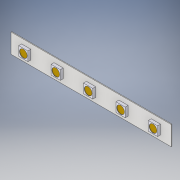
# Autodesk Inventor part: LEDStrip 5x
Saved by Autodesk Inventor 2019 (Build 230136000, 136)
## iProperties
Created: 2022-03-28
Part Number: LEDStrip 5x
Material: Generic
Document SubType Name: Modeling
Designer: Lix
Density: 1 g/cm^3
Appearance: Default
Author: Lix
Autodesk Inventor part; units mm, degrees
ref_plane "YZ Plane" through (0, 0, 0) normal (1, 0, 0) x (0, 1, 0)
ref_plane "XZ Plane" through (0, 0, 0) normal (0, 1, 0) x (-1, 0, 0)
ref_plane "XY Plane" through (0, 0, 0) normal (0, 0, 1) x (1, 0, 0)
sketch "Sketch1" plane through (0, 0, 0) normal (0, 0, 1) x (1, 0, 0)
  line L0 (-41.5, 5) -> (41.5, 5)
  line L1 (41.5, 5) -> (41.5, -5)
  line L2 (41.5, -5) -> (-41.5, -5)
  line L3 (-41.5, -5) -> (-41.5, 5)
  line L4 (-41.5, 5) -> (41.5, -5) construction
  line L5 (41.5, 5) -> (-41.5, -5) construction
  point P0 (0, 0)
  dimension "d0" = 83
  dimension "d1" = 10
  constraints: 12 end point, 2 midpoint, 2 parallel, 1 horizontal, 1 perpendicular
  measures "d0" distance of L1.end L2.end
  measures "d1" distance of L0.end L1.end
extrude "Extrusion1" add sketch "Sketch1" along normal blind 0.4
sketch "Sketch2" plane through (0, 0, 0.4) normal (0, 0, 1) x (1, 0, 0)
  line L0 (31.2, 2.4) -> (36, 2.4)
  line L1 (36, 2.4) -> (36, -2.4)
  line L2 (36, -2.4) -> (31.2, -2.4)
  line L3 (31.2, -2.4) -> (31.2, 2.4)
  line L4 (31.2, 2.4) -> (36, -2.4) construction
  line L5 (36, 2.4) -> (31.2, -2.4) construction
  line L6 (-41.5, 5) -> (-41.5, -5) projected
  line L7 (41.5, -5) -> (41.5, 5) projected
  line L8 (14.4, 2.4) -> (19.2, 2.4)
  line L9 (19.2, 2.4) -> (19.2, -2.4)
  line L10 (19.2, -2.4) -> (14.4, -2.4)
  line L11 (14.4, -2.4) -> (14.4, 2.4)
  line L12 (14.4, 2.4) -> (19.2, -2.4) construction
  line L13 (19.2, 2.4) -> (14.4, -2.4) construction
  line L14 (-2.4, 2.4) -> (2.4, 2.4)
  line L15 (2.4, 2.4) -> (2.4, -2.4)
  line L16 (2.4, -2.4) -> (-2.4, -2.4)
  line L17 (-2.4, -2.4) -> (-2.4, 2.4)
  line L18 (-2.4, 2.4) -> (2.4, -2.4) construction
  line L19 (2.4, 2.4) -> (-2.4, -2.4) construction
  line L20 (-19.2, 2.4) -> (-14.4, 2.4)
  line L21 (-14.4, 2.4) -> (-14.4, -2.4)
  line L22 (-14.4, -2.4) -> (-19.2, -2.4)
  line L23 (-19.2, -2.4) -> (-19.2, 2.4)
  line L24 (-19.2, 2.4) -> (-14.4, -2.4) construction
  line L25 (-14.4, 2.4) -> (-19.2, -2.4) construction
  line L26 (-36, 2.4) -> (-31.2, 2.4)
  line L27 (-31.2, 2.4) -> (-31.2, -2.4)
  line L28 (-31.2, -2.4) -> (-36, -2.4)
  line L29 (-36, -2.4) -> (-36, 2.4)
  line L30 (-36, 2.4) -> (-31.2, -2.4) construction
  line L31 (-31.2, 2.4) -> (-36, -2.4) construction
  point P0 (0, 0)
  point P1 (33.6, 0)
  point P2 (33.6, 0)
  point P3 (-41.5, 0)
  point P4 (16.8, 0)
  point P5 (16.8, 0)
  point P6 (0, 0)
  point P7 (0, 0)
  point P8 (-16.8, 0)
  point P9 (-16.8, 0)
  point P10 (-33.6, 0)
  point P11 (-33.6, 0)
  dimension "d4" = 4.8
  dimension "d5" = 4.8
  dimension "d6" = 5.5
  dimension "d9" = 16.8
  constraints: 60 end point, 12 midpoint, 2 horizontal, 2 parallel, 1 collinear, 1 horizontal alignment, 1 perpendicular, 47 other
  measures "d4" distance of L1.end L2.end
  measures "d5" distance of L0.end L1.end
  measures "d6" distance between parallel lines of L7 L1
  measures "d9" distance of L0.start L8.start
extrude "Extrusion2" add sketch "Sketch2" along normal blind 1.5
sketch "Sketch3" plane through (0, 0, 1.9) normal (0, 0, 1) x (1, 0, 0)
  circle A0 centre (33.6, 0) radius 2
  line L0 (36, -2.4) -> (36, 2.4) projected
  line L1 (36, 2.4) -> (31.2, 2.4) projected
  point P0 (0, 0)
  point P1 (36, 0)
  point P2 (33.6, 2.4)
  dimension "d16" = 4
  constraints: 2 midpoint, 1 centre point, 1 horizontal alignment, 1 vertical alignment
  measures "d16" diameter of A0
extrude "Extrusion3" cut sketch "Sketch3" against normal blind 0.2
pattern_linear "Rectangular Pattern1" count 5 spacing 16.8 along (-1, 0, 0) of "Extrusion3"
body "Solid1"
